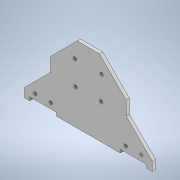
# Autodesk Inventor part: дно
Saved by Autodesk Inventor 2020 (Build 240168000, 168)
## iProperties
Created: 2025-01-24
Part Number: дно
Material: Типовые
Document SubType Name: Modeling
Designer: frozj
Density: 1 g/cm^3
Appearance: По умолчанию
Author: frozj
Autodesk Inventor part; units mm, degrees
ref_plane "YZ Plane" through (0, 0, 0) normal (1, 0, 0) x (0, 1, 0)
ref_plane "XZ Plane" through (0, 0, 0) normal (0, 1, 0) x (-1, 0, 0)
ref_plane "XY Plane" through (0, 0, 0) normal (0, 0, 1) x (1, 0, 0)
sketch "Эскиз1" plane through (0, 0, 0) normal (0, 0, 1) x (1, 0, 0)
  line L0 (57.5, -31.5) -> (-57.5, -31.5)
  line L1 (-57.5, -31.5) -> (-57.5, 31.5)
  line L2 (-57.5, 31.5) -> (57.5, 31.5)
  line L3 (57.5, 31.5) -> (57.5, -31.5)
  line L4 (57.5, -31.5) -> (-57.5, 31.5) construction
  line L5 (-57.5, -31.5) -> (57.5, 31.5) construction
  line L6 (0, 0) -> (0, 31.5)
  line L7 (0, 31.5) -> (12, 31.5)
  line L8 (12, 31.5) -> (12, 21.5)
  line L9 (12, 21.5) -> (0, 21.5)
  line L10 (0, 21.5) -> (0, 31.5)
  line L11 (0, 31.5) -> (-12, 31.5)
  line L12 (-12, 31.5) -> (-12, 21.5)
  line L13 (-12, 21.5) -> (0, 21.5)
  line L14 (0, 21.5) -> (0, 31.5)
  circle A0 centre (-12, 21.5) radius 1.5
  circle A1 centre (12, 21.5) radius 1.5
  line L15 (0, 0) -> (-33.75, 0)
  line L16 (-33.75, 0) -> (-33.75, -31.5)
  line L17 (-33.75, -31.5) -> (0, -31.5)
  line L18 (0, -31.5) -> (0, 0)
  line L19 (0, -31.5) -> (-33.75, -31.5)
  line L20 (-33.75, -31.5) -> (-33.75, -23.5)
  line L21 (-33.75, -23.5) -> (0, -23.5)
  line L22 (0, -23.5) -> (0, -31.5)
  line L23 (-57.5, -31.5) -> (57.5, -31.5)
  line L24 (57.5, -31.5) -> (57.5, -28.5)
  line L25 (57.5, -28.5) -> (-57.5, -28.5)
  line L26 (-57.5, -28.5) -> (-57.5, -31.5)
  circle A2 centre (-33.75, -23.5) radius 1.5
  line L27 (-33.75, -23.5) -> (-47.75, -23.5)
  line L28 (-47.75, -23.5) -> (-47.75, -31.5)
  line L29 (-47.75, -31.5) -> (-33.75, -31.5)
  line L30 (-33.75, -31.5) -> (-33.75, -23.5)
  circle A3 centre (-47.75, -23.5) radius 1.5
  line L31 (33.75, -31.5) -> (33.75, -23.5)
  circle A4 centre (33.75, -23.5) radius 1.5
  line L32 (47.75, -23.5) -> (47.75, -31.5)
  circle A5 centre (47.75, -23.5) radius 1.5
  line L33 (0, 0) -> (11.5, 0)
  circle A6 centre (11.5, 0) radius 1.5
  circle A7 centre (-11.5, 0) radius 1.5
  line L34 (-33.75, -31.5) -> (-28.75, -31.5)
  line L35 (-28.75, -31.5) -> (-28.75, -28.5)
  line L36 (-28.75, -28.5) -> (-33.75, -28.5)
  line L37 (-33.75, -28.5) -> (-33.75, -31.5)
  line L38 (-47.75, -31.5) -> (-52.75, -31.5)
  line L39 (-52.75, -31.5) -> (-52.75, -28.5)
  line L40 (-52.75, -28.5) -> (-47.75, -28.5)
  line L41 (-47.75, -28.5) -> (-47.75, -31.5)
  line L42 (28.75, -31.5) -> (28.75, -28.5)
  line L43 (52.75, -31.5) -> (52.75, -28.5)
  line L44 (-47.75, -23.5) -> (-57.5, -23.5)
  line L45 (-57.5, -23.5) -> (-34, 0)
  line L46 (-57.5, -23.5) -> (-24.266, -23.5) construction
  line L47 (-12, 31.5) -> (-34, 9.5)
  line L48 (-12, 31.5) -> (19.1127, 31.5) construction
  line L49 (-34, 9.5) -> (-34, 0)
  line L50 (-57.5, -31.5) -> (57.5, 31.5) construction
  line L51 (57.5, -23.5) -> (34, 0)
  line L52 (12, 31.5) -> (34, 9.5)
  line L53 (34, 9.5) -> (34, 0)
  line L54 (34, 9.5) -> (34, 31.5)
  line L55 (-34, 9.5) -> (-34, 31.5)
  line L56 (12, 31.5) -> (15, 31.5)
  line L57 (15, 31.5) -> (34, 12.5)
  line L58 (-12, 31.5) -> (-15, 31.5)
  line L59 (-15, 31.5) -> (-34, 12.5)
  line L60 (-57.5, 31.5) -> (57.5, 31.5)
  line L61 (57.5, 31.5) -> (57.5, 36.5)
  line L62 (57.5, 36.5) -> (-57.5, 36.5)
  line L63 (-57.5, 36.5) -> (-57.5, 31.5)
  line L64 (-15, 31.5) -> (-10, 36.5)
  line L65 (15, 31.5) -> (10, 36.5)
  point P0 (-47.75, -28.5)
  point P1 (-33.75, -28.5)
  point P2 (33.75, -28.5)
  point P3 (47.75, -28.5)
  dimension "d0" = 115
  dimension "d1" = 63
  dimension "d2" = 12
  dimension "d3" = 10
  dimension "d4" = 12
  dimension "d5" = 3
  dimension "d6" = 3
  dimension "d7" = 33.75
  dimension "d8" = 8
  dimension "d9" = 3
  dimension "d10" = 3
  dimension "d11" = 14
  dimension "d12" = 3
  dimension "d13" = 11.5
  dimension "d14" = 3
  dimension "d17" = 5
  dimension "d18" = 5
  dimension "d19" = 45
  dimension "d20" = 135
  dimension "d21" = 3
  dimension "d22" = 135
  dimension "d23" = 3
  dimension "d24" = 5
  constraints: 132 end point, 21 parallel, 17 point on line, 16 symmetric about line, 15 perpendicular, 12 horizontal, 8 centre point, 7 coincident, 3 midpoint, 2 equal length, 3 other
  measures "d0" distance of L1.end L2.end
  measures "d1" distance of L0.end L1.end
  measures "d2" distance of L8.end L9.end
  measures "d3" distance of L7.end L8.end
  measures "d4" distance of L13.end L12.end
  measures "d5" diameter of A0
  measures "d6" diameter of A1
  measures "d7" distance of L17.end L16.end
  measures "d8" distance of L19.end L20.end
  measures "d9" distance of L24.end L23.end
  measures "d10" diameter of A2
  measures "d11" distance of L29.end L28.end
  measures "d12" diameter of A3
  measures "d13" distance of L6.start L33.end
  measures "d14" diameter of A6
  measures "d17" distance of L36.end L35.end
  measures "d18" distance of L39.end L40.end
  measures "d19" angle of L46 L45
  measures "d20" angle of L47 L48
  measures "d21" distance of L7.end L56.end
  measures "d22" angle of L56 L57
  measures "d23" distance of L11.end L58.end
  measures "d24" distance of L61.end L60.end
extrude "Выдавливание1" add sketch "Эскиз1" along normal blind 3 contours L0 L43 L25 L3 | L25 L18 L6 L9 A1 L8 L52 L53 L51 L3 | L0 L18 L25 L42 | L52 L2 L57 L54 | L0 L35 L25 L18 | L2 L64 L62 L65 | L8 A1 L9 L6 L2 | L25 L16 A2 L21 L18 | L6 L13 A0 L12 L2 | L21 A2 L16 L15 A7 L18 | L2 L47 L55 L59 | L12 A0 L13 L6 L15 A7 L16 A2 L27 A3 L44 L45 L49 L47 | L25 L28 A3 L27 A2 L16 | L0 L1 L25 L39 | L25 L1 L44 A3 L28
